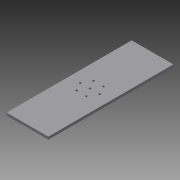
# Autodesk Inventor part: Claw Plate
Saved by Autodesk Inventor 2014 (Build 180170000, 170)
## iProperties
Created: 2015-01-25
Part Number: Claw Plate
Material: Generic
Document SubType Name: Modeling
Designer: chappelled
Density: 1 g/cm^3
Appearance: Default
Author: chappelled
Autodesk Inventor part; units mm, degrees
ref_plane "YZ Plane" through (0, 0, 0) normal (1, 0, 0) x (0, 1, 0)
ref_plane "XZ Plane" through (0, 0, 0) normal (0, 1, 0) x (-1, 0, 0)
ref_plane "XY Plane" through (0, 0, 0) normal (0, 0, 1) x (1, 0, 0)
sketch "Sketch1" plane through (0, 0, 0) normal (0, 1, 0) x (-1, 0, 0)
  line L0 (0, 0) -> (-101.6, 0)
  line L1 (-101.6, 0) -> (-101.6, 304.8)
  line L2 (-101.6, 304.8) -> (0, 304.8)
  line L3 (0, 304.8) -> (0, 0)
  point P0 (-50.8, 152.4)
  dimension "d0" = 101.6
  dimension "d1" = 304.8
  dimension "d25" = 50.8
  dimension "d26" = 152.4
  constraints: 8 end point, 2 parallel, 1 horizontal, 1 perpendicular
  measures "d0" distance of L1.end L2.end
  measures "d1" distance of L0.end L1.end
  measures "d25" distance from line of L3 point (-50.8, 152.4)
  measures "d26" distance from line of L0 point (-50.8, 152.4)
extrude "Extrusion1" add sketch "Sketch1" along normal blind 6.35
hole "Hole2" at (26.9875, 6.35, 152.4) direction (0, -1, 0) diameter 4.8768 end through all
hole "Hole3" at (50.8, 6.35, 152.4) direction (0, -1, 0) diameter 4.8768 end through all
pattern_circular "Circular Pattern2" count 6 over 360 about axis through (50.8, -315.0002, 152.4) along (0, 1, 0) of "Hole2"
body "Solid1"
